Autodesk Fusion 360 part; units mm, degrees
note: some values were not read from the file. Set by a fixed rule: which sketch regions a step uses.
(part 16 of 20)
  spline S91 degree 5 poles (-29.6298, 9.1146) (-29.6276, 9.1129) (-29.6234, 9.1096) (-29.6169, 9.1047) (-29.6084, 9.0981) (-29.5977, 9.09) (-29.587, 9.0818) (-29.5763, 9.0737) (-29.5657, 9.0657) (-29.555, 9.0576) (-29.5444, 9.0496) (-29.5338, 9.0416) (-29.5232, 9.0337) (-29.5127, 9.0258) (-29.5021, 9.0179) (-29.4915, 9.0101) (-29.481, 9.0022) (-29.4705, 8.9945) (-29.46, 8.9867) (-29.4495, 8.979) (-29.4391, 8.9713) (-29.4286, 8.9637) (-29.4182, 8.956) (-29.4078, 8.9485) (-29.3974, 8.9409) (-29.387, 8.9334) (-29.3766, 8.9259) (-29.3663, 8.9184) (-29.356, 8.911) (-29.3457, 8.9036) (-29.3354, 8.8963) (-29.3251, 8.8889) (-29.3148, 8.8816) (-29.3046, 8.8744) (-29.2944, 8.8671) (-29.2842, 8.86) (-29.274, 8.8528) (-29.2638, 8.8457) (-29.2537, 8.8386) (-29.2435, 8.8315) (-29.2334, 8.8245) (-29.2233, 8.8175) (-29.2132, 8.8105) (-29.2032, 8.8036) (-29.1932, 8.7967) (-29.1831, 8.7898) (-29.1731, 8.783) (-29.1632, 8.7762) (-29.1532, 8.7694) (-29.1433, 8.7626) (-29.1334, 8.7559) (-29.1235, 8.7493) (-29.1136, 8.7426) (-29.1037, 8.736) (-29.0939, 8.7295) (-29.0841, 8.7229) (-29.0743, 8.7164) (-29.0646, 8.7099) (-29.0548, 8.7035) (-29.0451, 8.6971) (-29.0354, 8.6907) (-29.0257, 8.6844) (-29.016, 8.6781) (-29.0064, 8.6718) (-28.9968, 8.6656) (-28.9872, 8.6593) (-28.9776, 8.6532) (-28.9681, 8.647) (-28.9586, 8.6409) (-28.9491, 8.6348) (-28.9396, 8.6288) (-28.9302, 8.6228) (-28.9207, 8.6168) (-28.9113, 8.6109) (-28.902, 8.605) (-28.8926, 8.5991) (-28.8833, 8.5932) (-28.874, 8.5874) (-28.8647, 8.5817) (-28.8555, 8.5759) (-28.8462, 8.5702) (-28.837, 8.5645) (-28.8279, 8.5589) (-28.8187, 8.5533) (-28.8096, 8.5477) (-28.8005, 8.5422) (-28.7914, 8.5367) (-28.7824, 8.5312) (-28.7734, 8.5257) (-28.7644, 8.5203) (-28.7554, 8.515) (-28.7465, 8.5096) (-28.7376, 8.5043) (-28.7287, 8.499) (-28.7199, 8.4938) (-28.711, 8.4886) (-28.7022, 8.4834) (-28.6935, 8.4783) (-28.6847, 8.4732) (-28.676, 8.4681) (-28.6674, 8.463) (-28.6587, 8.458) (-28.6501, 8.4531) (-28.6415, 8.4481) (-28.633, 8.4432) (-28.6244, 8.4384) (-28.616, 8.4335) (-28.6075, 8.4287) (-28.5991, 8.4239) (-28.5907, 8.4192) (-28.5823, 8.4145) (-28.574, 8.4098) (-28.5657, 8.4052) (-28.5574, 8.4006) (-28.5491, 8.396) (-28.5409, 8.3915) (-28.5328, 8.387) (-28.5246, 8.3825) (-28.5165, 8.3781) (-28.5085, 8.3737) (-28.5004, 8.3693) (-28.4924, 8.365) (-28.4845, 8.3607) (-28.4765, 8.3565) (-28.4686, 8.3522) (-28.4608, 8.348) (-28.4529, 8.3439) (-28.4452, 8.3398) (-28.4374, 8.3357) (-28.4297, 8.3316) (-28.422, 8.3276) (-28.4144, 8.3236) (-28.4068, 8.3196) (-28.3992, 8.3157) (-28.3917, 8.3118) (-28.3842, 8.308) (-28.3767, 8.3042) (-28.3693, 8.3004) (-28.3619, 8.2966) (-28.3546, 8.2929) (-28.3473, 8.2892) (-28.3401, 8.2856) (-28.3329, 8.282) (-28.3257, 8.2784) (-28.3186, 8.2748) (-28.3115, 8.2713) (-28.3044, 8.2678) (-28.2974, 8.2644) (-28.2905, 8.261) (-28.2835, 8.2576) (-28.2767, 8.2543) (-28.2698, 8.251) (-28.263, 8.2477) (-28.2563, 8.2445) (-28.2496, 8.2412) (-28.2429, 8.2381) (-28.2363, 8.2349) (-28.2298, 8.2318) (-28.2233, 8.2288) (-28.2168, 8.2257) (-28.2104, 8.2227) (-28.204, 8.2198) (-28.1977, 8.2169) (-28.1914, 8.214) (-28.1851, 8.2111) (-28.179, 8.2083) (-28.1728, 8.2055) (-28.1667, 8.2027) (-28.1607, 8.2) (-28.1547, 8.1973) (-28.1488, 8.1947) (-28.1429, 8.192) (-28.1371, 8.1895) (-28.1313, 8.1869) (-28.1256, 8.1844) (-28.1199, 8.1819) (-28.1143, 8.1795) (-28.1087, 8.177) (-28.1032, 8.1747) (-28.0978, 8.1723) (-28.0924, 8.17) (-28.087, 8.1677) (-28.0818, 8.1655) (-28.0765, 8.1633) (-28.0714, 8.1611) (-28.0663, 8.159) (-28.0612, 8.1569) (-28.0562, 8.1548) (-28.0513, 8.1528) (-28.0464, 8.1508) (-28.0416, 8.1488) (-28.0369, 8.1469) (-28.0322, 8.145) (-28.0276, 8.1432) (-28.023, 8.1413) (-28.0185, 8.1395) (-28.0141, 8.1378) (-28.0097, 8.1361) (-28.0054, 8.1344) (-28.0012, 8.1327) (-27.997, 8.1311) (-27.9929, 8.1295) (-27.9889, 8.128) (-27.9849, 8.1265) (-27.9811, 8.125) (-27.9772, 8.1236) (-27.9735, 8.1222) (-27.9698, 8.1208) (-27.9662, 8.1194) (-27.9627, 8.1181) (-27.9593, 8.1169) (-27.9559, 8.1156) (-27.9526, 8.1144) (-27.9494, 8.1133) (-27.9462, 8.1121) (-27.9432, 8.1111) (-27.9402, 8.11) (-27.9373, 8.109) (-27.9345, 8.108) (-27.9318, 8.107) (-27.9291, 8.1061) (-27.9265, 8.1052) (-27.9241, 8.1044) (-27.9217, 8.1036) (-27.9194, 8.1028) (-27.9172, 8.102) (-27.915, 8.1013) (-27.913, 8.1007) (-27.9111, 8.1) (-27.9092, 8.0994) (-27.9075, 8.0988) (-27.9058, 8.0983) (-27.9043, 8.0978) (-27.9028, 8.0973) (-27.9015, 8.0969) (-27.9002, 8.0965) (-27.8991, 8.0962) (-27.898, 8.0958) (-27.8971, 8.0956) (-27.8963, 8.0953) (-27.8956, 8.0951) (-27.8951, 8.0949) (-27.8948, 8.0948) (-27.8946, 8.0948) (-27.8945, 8.0948) knots -1 -1 -1 -1 -1 -1 -0.99583333 -0.99166667 -0.9875 -0.98333333 -0.97916667 -0.975 -0.97083333 -0.96666667 -0.9625 -0.95833333 -0.95416667 -0.95 -0.94583333 -0.94166667 -0.9375 -0.93333333 -0.92916667 -0.925 -0.92083333 -0.91666667 -0.9125 -0.90833333 -0.90416667 -0.9 -0.89583333 -0.89166667 -0.8875 -0.88333333 -0.87916667 -0.875 -0.87083333 -0.86666667 -0.8625 -0.85833333 -0.85416667 -0.85 -0.84583333 -0.84166667 -0.8375 -0.83333333 -0.82916667 -0.825 -0.82083333 -0.81666667 -0.8125 -0.80833333 -0.80416667 -0.8 -0.79583333 -0.79166667 -0.7875 -0.78333333 -0.77916667 -0.775 -0.77083333 -0.76666667 -0.7625 -0.75833333 -0.75416667 -0.75 -0.74583333 -0.74166667 -0.7375 -0.73333333 -0.72916667 -0.725 -0.72083333 -0.71666667 -0.7125 -0.70833333 -0.70416667 -0.7 -0.69583333 -0.69166667 -0.6875 -0.68333333 -0.67916667 -0.675 -0.67083333 -0.66666667 -0.6625 -0.65833333 -0.65416667 -0.65 -0.64583333 -0.64166667 -0.6375 -0.63333333 -0.62916667 -0.625 -0.62083333 -0.61666667 -0.6125 -0.60833333 -0.60416667 -0.6 -0.59583333 -0.59166667 -0.5875 -0.58333333 -0.57916667 -0.575 -0.57083333 -0.56666667 -0.5625 -0.55833333 -0.55416667 -0.55 -0.54583333 -0.54166667 -0.5375 -0.53333333 -0.52916667 -0.525 -0.52083333 -0.51666667 -0.5125 -0.50833333 -0.50416667 -0.5 -0.49583333 -0.49166667 -0.4875 -0.48333333 -0.47916667 -0.475 -0.47083333 -0.46666667 -0.4625 -0.45833333 -0.45416667 -0.45 -0.44583333 -0.44166667 -0.4375 -0.43333333 -0.42916667 -0.425 -0.42083333 -0.41666667 -0.4125 -0.40833333 -0.40416667 -0.4 -0.39583333 -0.39166667 -0.3875 -0.38333333 -0.37916667 -0.375 -0.37083333 -0.36666667 -0.3625 -0.35833333 -0.35416667 -0.35 -0.34583333 -0.34166667 -0.3375 -0.33333333 -0.32916667 -0.325 -0.32083333 -0.31666667 -0.3125 -0.30833333 -0.30416667 -0.3 -0.29583333 -0.29166667 -0.2875 -0.28333333 -0.27916667 -0.275 -0.27083333 -0.26666667 -0.2625 -0.25833333 -0.25416667 -0.25 -0.24583333 -0.24166667 -0.2375 -0.23333333 -0.22916667 -0.225 -0.22083333 -0.21666667 -0.2125 -0.20833333 -0.20416667 -0.2 -0.19583333 -0.19166667 -0.1875 -0.18333333 -0.17916667 -0.175 -0.17083333 -0.16666667 -0.1625 -0.15833333 -0.15416667 -0.15 -0.14583333 -0.14166667 -0.1375 -0.13333333 -0.12916667 -0.125 -0.12083333 -0.11666667 -0.1125 -0.10833333 -0.10416667 -0.1 -0.09583333 -0.09166667 -0.0875 -0.08333333 -0.07916667 -0.075 -0.07083333 -0.06666667 -0.0625 -0.05833333 -0.05416667 -0.05 -0.04583333 -0.04166667 -0.0375 -0.03333333 -0.02916667 -0.025 -0.02083333 -0.01666667 -0.0125 -0.00833333 -0.00416667 0 0 0 0 0 0
  line L187 (-26.8955, 10.9662) -> (-26.8948, 10.9659)
  arc A90 (5.0824, 28.2972) -> (3.9106, 28.4828) centre (0, 0) ccw
  line L188 (-25.8803, 12.5209) -> (-26.1453, 12.6491)
  arc A91 (6.9214, 30.2174) -> (5.9675, 30.4202) centre (0, 0) ccw
  arc A92 (8.0125, 27.6109) -> (6.8665, 27.918) centre (0, 0) ccw
  line L189 (5.1345, 28.587) -> (5.0824, 28.2972)
  spline S92 degree 5 poles (9.1146, 29.6298) (9.1129, 29.6276) (9.1096, 29.6234) (9.1047, 29.6169) (9.0981, 29.6084) (9.09, 29.5977) (9.0818, 29.587) (9.0737, 29.5763) (9.0657, 29.5657) (9.0576, 29.555) (9.0496, 29.5444) (9.0416, 29.5338) (9.0337, 29.5232) (9.0258, 29.5127) (9.0179, 29.5021) (9.0101, 29.4915) (9.0022, 29.481) (8.9945, 29.4705) (8.9867, 29.46) (8.979, 29.4495) (8.9713, 29.4391) (8.9637, 29.4286) (8.956, 29.4182) (8.9485, 29.4078) (8.9409, 29.3974) (8.9334, 29.387) (8.9259, 29.3766) (8.9184, 29.3663) (8.911, 29.356) (8.9036, 29.3457) (8.8963, 29.3354) (8.8889, 29.3251) (8.8816, 29.3148) (8.8744, 29.3046) (8.8671, 29.2944) (8.86, 29.2842) (8.8528, 29.274) (8.8457, 29.2638) (8.8386, 29.2537) (8.8315, 29.2435) (8.8245, 29.2334) (8.8175, 29.2233) (8.8105, 29.2132) (8.8036, 29.2032) (8.7967, 29.1932) (8.7898, 29.1831) (8.783, 29.1731) (8.7762, 29.1632) (8.7694, 29.1532) (8.7626, 29.1433) (8.7559, 29.1334) (8.7493, 29.1235) (8.7426, 29.1136) (8.736, 29.1037) (8.7295, 29.0939) (8.7229, 29.0841) (8.7164, 29.0743) (8.7099, 29.0646) (8.7035, 29.0548) (8.6971, 29.0451) (8.6907, 29.0354) (8.6844, 29.0257) (8.6781, 29.016) (8.6718, 29.0064) (8.6656, 28.9968) (8.6593, 28.9872) (8.6532, 28.9776) (8.647, 28.9681) (8.6409, 28.9586) (8.6348, 28.9491) (8.6288, 28.9396) (8.6228, 28.9302) (8.6168, 28.9207) (8.6109, 28.9113) (8.605, 28.902) (8.5991, 28.8926) (8.5932, 28.8833) (8.5874, 28.874) (8.5817, 28.8647) (8.5759, 28.8555) (8.5702, 28.8462) (8.5645, 28.837) (8.5589, 28.8279) (8.5533, 28.8187) (8.5477, 28.8096) (8.5422, 28.8005) (8.5367, 28.7914) (8.5312, 28.7824) (8.5257, 28.7734) (8.5203, 28.7644) (8.515, 28.7554) (8.5096, 28.7465) (8.5043, 28.7376) (8.499, 28.7287) (8.4938, 28.7199) (8.4886, 28.711) (8.4834, 28.7022) (8.4783, 28.6935) (8.4732, 28.6847) (8.4681, 28.676) (8.463, 28.6674) (8.458, 28.6587) (8.4531, 28.6501) (8.4481, 28.6415) (8.4432, 28.633) (8.4384, 28.6244) (8.4335, 28.616) (8.4287, 28.6075) (8.4239, 28.5991) (8.4192, 28.5907) (8.4145, 28.5823) (8.4098, 28.574) (8.4052, 28.5657) (8.4006, 28.5574) (8.396, 28.5491) (8.3915, 28.5409) (8.387, 28.5328) (8.3825, 28.5246) (8.3781, 28.5165) (8.3737, 28.5085) (8.3693, 28.5004) (8.365, 28.4924) (8.3607, 28.4845) (8.3565, 28.4765) (8.3522, 28.4686) (8.348, 28.4608) (8.3439, 28.4529) (8.3398, 28.4452) (8.3357, 28.4374) (8.3316, 28.4297) (8.3276, 28.422) (8.3236, 28.4144) (8.3196, 28.4068) (8.3157, 28.3992) (8.3118, 28.3917) (8.308, 28.3842) (8.3042, 28.3767) (8.3004, 28.3693) (8.2966, 28.3619) (8.2929, 28.3546) (8.2892, 28.3473) (8.2856, 28.3401) (8.282, 28.3329) (8.2784, 28.3257) (8.2748, 28.3186) (8.2713, 28.3115) (8.2678, 28.3044) (8.2644, 28.2974) (8.261, 28.2905) (8.2576, 28.2835) (8.2543, 28.2767) (8.251, 28.2698) (8.2477, 28.263) (8.2445, 28.2563) (8.2412, 28.2496) (8.2381, 28.2429) (8.2349, 28.2363) (8.2318, 28.2298) (8.2288, 28.2233) (8.2257, 28.2168) (8.2227, 28.2104) (8.2198, 28.204) (8.2169, 28.1977) (8.214, 28.1914) (8.2111, 28.1851) (8.2083, 28.179) (8.2055, 28.1728) (8.2027, 28.1667) (8.2, 28.1607) (8.1973, 28.1547) (8.1947, 28.1488) (8.192, 28.1429) (8.1895, 28.1371) (8.1869, 28.1313) (8.1844, 28.1256) (8.1819, 28.1199) (8.1795, 28.1143) (8.177, 28.1087) (8.1747, 28.1032) (8.1723, 28.0978) (8.17, 28.0924) (8.1677, 28.087) (8.1655, 28.0818) (8.1633, 28.0765) (8.1611, 28.0714) (8.159, 28.0663) (8.1569, 28.0612) (8.1548, 28.0562) (8.1528, 28.0513) (8.1508, 28.0464) (8.1488, 28.0416) (8.1469, 28.0369) (8.145, 28.0322) (8.1432, 28.0276) (8.1413, 28.023) (8.1395, 28.0185) (8.1378, 28.0141) (8.1361, 28.0097) (8.1344, 28.0054) (8.1327, 28.0012) (8.1311, 27.997) (8.1295, 27.9929) (8.128, 27.9889) (8.1265, 27.9849) (8.125, 27.9811) (8.1236, 27.9772) (8.1222, 27.9735) (8.1208, 27.9698) (8.1194, 27.9662) (8.1181, 27.9627) (8.1169, 27.9593) (8.1156, 27.9559) (8.1144, 27.9526) (8.1133, 27.9494) (8.1121, 27.9462) (8.1111, 27.9432) (8.11, 27.9402) (8.109, 27.9373) (8.108, 27.9345) (8.107, 27.9318) (8.1061, 27.9291) (8.1052, 27.9265) (8.1044, 27.9241) (8.1036, 27.9217) (8.1028, 27.9194) (8.102, 27.9172) (8.1013, 27.915) (8.1007, 27.913) (8.1, 27.9111) (8.0994, 27.9092) (8.0988, 27.9075) (8.0983, 27.9058) (8.0978, 27.9043) (8.0973, 27.9028) (8.0969, 27.9015) (8.0965, 27.9002) (8.0962, 27.8991) (8.0958, 27.898) (8.0956, 27.8971) (8.0953, 27.8963) (8.0951, 27.8956) (8.0949, 27.8951) (8.0948, 27.8948) (8.0948, 27.8946) (8.0948, 27.8945) knots -1 -1 -1 -1 -1 -1 -0.99583333 -0.99166667 -0.9875 -0.98333333 -0.97916667 -0.975 -0.97083333 -0.96666667 -0.9625 -0.95833333 -0.95416667 -0.95 -0.94583333 -0.94166667 -0.9375 -0.93333333 -0.92916667 -0.925 -0.92083333 -0.91666667 -0.9125 -0.90833333 -0.90416667 -0.9 -0.89583333 -0.89166667 -0.8875 -0.88333333 -0.87916667 -0.875 -0.87083333 -0.86666667 -0.8625 -0.85833333 -0.85416667 -0.85 -0.84583333 -0.84166667 -0.8375 -0.83333333 -0.82916667 -0.825 -0.82083333 -0.81666667 -0.8125 -0.80833333 -0.80416667 -0.8 -0.79583333 -0.79166667 -0.7875 -0.78333333 -0.77916667 -0.775 -0.77083333 -0.76666667 -0.7625 -0.75833333 -0.75416667 -0.75 -0.74583333 -0.74166667 -0.7375 -0.73333333 -0.72916667 -0.725 -0.72083333 -0.71666667 -0.7125 -0.70833333 -0.70416667 -0.7 -0.69583333 -0.69166667 -0.6875 -0.68333333 -0.67916667 -0.675 -0.67083333 -0.66666667 -0.6625 -0.65833333 -0.65416667 -0.65 -0.64583333 -0.64166667 -0.6375 -0.63333333 -0.62916667 -0.625 -0.62083333 -0.61666667 -0.6125 -0.60833333 -0.60416667 -0.6 -0.59583333 -0.59166667 -0.5875 -0.58333333 -0.57916667 -0.575 -0.57083333 -0.56666667 -0.5625 -0.55833333 -0.55416667 -0.55 -0.54583333 -0.54166667 -0.5375 -0.53333333 -0.52916667 -0.525 -0.52083333 -0.51666667 -0.5125 -0.50833333 -0.50416667 -0.5 -0.49583333 -0.49166667 -0.4875 -0.48333333 -0.47916667 -0.475 -0.47083333 -0.46666667 -0.4625 -0.45833333 -0.45416667 -0.45 -0.44583333 -0.44166667 -0.4375 -0.43333333 -0.42916667 -0.425 -0.42083333 -0.41666667 -0.4125 -0.40833333 -0.40416667 -0.4 -0.39583333 -0.39166667 -0.3875 -0.38333333 -0.37916667 -0.375 -0.37083333 -0.36666667 -0.3625 -0.35833333 -0.35416667 -0.35 -0.34583333 -0.34166667 -0.3375 -0.33333333 -0.32916667 -0.325 -0.32083333 -0.31666667 -0.3125 -0.30833333 -0.30416667 -0.3 -0.29583333 -0.29166667 -0.2875 -0.28333333 -0.27916667 -0.275 -0.27083333 -0.26666667 -0.2625 -0.25833333 -0.25416667 -0.25 -0.24583333 -0.24166667 -0.2375 -0.23333333 -0.22916667 -0.225 -0.22083333 -0.21666667 -0.2125 -0.20833333 -0.20416667 -0.2 -0.19583333 -0.19166667 -0.1875 -0.18333333 -0.17916667 -0.175 -0.17083333 -0.16666667 -0.1625 -0.15833333 -0.15416667 -0.15 -0.14583333 -0.14166667 -0.1375 -0.13333333 -0.12916667 -0.125 -0.12083333 -0.11666667 -0.1125 -0.10833333 -0.10416667 -0.1 -0.09583333 -0.09166667 -0.0875 -0.08333333 -0.07916667 -0.075 -0.07083333 -0.06666667 -0.0625 -0.05833333 -0.05416667 -0.05 -0.04583333 -0.04166667 -0.0375 -0.03333333 -0.02916667 -0.025 -0.02083333 -0.01666667 -0.0125 -0.00833333 -0.00416667 0 0 0 0 0 0
  line L190 (-26.1453, 12.6491) -> (-26.1461, 12.6495)
  arc A93 (-27.6109, 8.0125) -> (-27.918, 6.8665) centre (0, 0) ccw
  line L191 (6.9368, 28.2039) -> (6.937, 28.2047)
  arc A94 (-10.8547, -26.6221) -> (-9.7471, -27.0473) centre (0, 0) ccw
  arc A95 (28.7355, 0.9119) -> (28.6734, 2.0967) centre (0, 0) ccw
  spline S93 degree 5 poles (-12.1618, -28.5147) (-12.16, -28.5128) (-12.1562, -28.5089) (-12.1506, -28.503) (-12.1432, -28.4951) (-12.134, -28.4854) (-12.1248, -28.4756) (-12.1156, -28.4658) (-12.1065, -28.4561) (-12.0973, -28.4464) (-12.0883, -28.4366) (-12.0792, -28.4269) (-12.0702, -28.4172) (-12.0613, -28.4075) (-12.0523, -28.3978) (-12.0434, -28.3882) (-12.0345, -28.3785) (-12.0257, -28.3689) (-12.0169, -28.3593) (-12.0081, -28.3496) (-11.9994, -28.34) (-11.9907, -28.3305) (-11.982, -28.3209) (-11.9734, -28.3113) (-11.9648, -28.3018) (-11.9562, -28.2922) (-11.9477, -28.2827) (-11.9392, -28.2732) (-11.9307, -28.2637) (-11.9223, -28.2542) (-11.9139, -28.2447) (-11.9055, -28.2353) (-11.8972, -28.2259) (-11.8889, -28.2164) (-11.8807, -28.207) (-11.8724, -28.1976) (-11.8643, -28.1882) (-11.8561, -28.1789) (-11.848, -28.1695) (-11.8399, -28.1602) (-11.8318, -28.1509) (-11.8238, -28.1416) (-11.8158, -28.1323) (-11.8079, -28.123) (-11.8, -28.1137) (-11.7921, -28.1045) (-11.7843, -28.0953) (-11.7765, -28.0861) (-11.7687, -28.0769) (-11.7609, -28.0677) (-11.7532, -28.0585) (-11.7456, -28.0494) (-11.7379, -28.0403) (-11.7303, -28.0312) (-11.7228, -28.0221) (-11.7153, -28.013) (-11.7078, -28.0039) (-11.7003, -27.9949) (-11.6929, -27.9859) (-11.6855, -27.9769) (-11.6781, -27.9679) (-11.6708, -27.9589) (-11.6635, -27.95) (-11.6563, -27.9411) (-11.6491, -27.9322) (-11.6419, -27.9233) (-11.6348, -27.9144) (-11.6276, -27.9055) (-11.6206, -27.8967) (-11.6135, -27.8879) (-11.6065, -27.8791) (-11.5996, -27.8704) (-11.5927, -27.8616) (-11.5858, -27.8529) (-11.5789, -27.8442) (-11.5721, -27.8355) (-11.5653, -27.8268) (-11.5585, -27.8182) (-11.5518, -27.8096) (-11.5452, -27.801) (-11.5385, -27.7924) (-11.5319, -27.7838) (-11.5253, -27.7753) (-11.5188, -27.7668) (-11.5123, -27.7583) (-11.5058, -27.7498) (-11.4994, -27.7414) (-11.493, -27.733) (-11.4867, -27.7246) (-11.4803, -27.7162) (-11.4741, -27.7078) (-11.4678, -27.6995) (-11.4616, -27.6912) (-11.4554, -27.6829) (-11.4493, -27.6747) (-11.4432, -27.6665) (-11.4371, -27.6582) (-11.4311, -27.6501) (-11.4251, -27.6419) (-11.4192, -27.6338) (-11.4132, -27.6257) (-11.4074, -27.6176) (-11.4015, -27.6096) (-11.3957, -27.6015) (-11.3899, -27.5936) (-11.3842, -27.5856) (-11.3785, -27.5776) (-11.3728, -27.5697) (-11.3672, -27.5618) (-11.3616, -27.554) (-11.3561, -27.5462) (-11.3506, -27.5384) (-11.3451, -27.5306) (-11.3396, -27.5228) (-11.3342, -27.5151) (-11.3289, -27.5074) (-11.3235, -27.4998) (-11.3183, -27.4922) (-11.313, -27.4846) (-11.3078, -27.477) (-11.3026, -27.4695) (-11.2975, -27.462) (-11.2924, -27.4545) (-11.2873, -27.447) (-11.2823, -27.4396) (-11.2773, -27.4323) (-11.2723, -27.4249) (-11.2674, -27.4176) (-11.2625, -27.4103) (-11.2577, -27.4031) (-11.2529, -27.3958) (-11.2481, -27.3887) (-11.2434, -27.3815) (-11.2387, -27.3744) (-11.234, -27.3673) (-11.2294, -27.3603) (-11.2248, -27.3533) (-11.2203, -27.3463) (-11.2158, -27.3393) (-11.2113, -27.3324) (-11.2069, -27.3256) (-11.2025, -27.3187) (-11.1982, -27.3119) (-11.1939, -27.3052) (-11.1896, -27.2985) (-11.1854, -27.2918) (-11.1812, -27.2851) (-11.177, -27.2785) (-11.1729, -27.272) (-11.1688, -27.2654) (-11.1648, -27.259) (-11.1608, -27.2525) (-11.1568, -27.2461) (-11.1529, -27.2397) (-11.149, -27.2334) (-11.1451, -27.2271) (-11.1413, -27.2209) (-11.1376, -27.2147) (-11.1338, -27.2085) (-11.1301, -27.2024) (-11.1265, -27.1963) (-11.1229, -27.1903) (-11.1193, -27.1843) (-11.1158, -27.1784) (-11.1123, -27.1725) (-11.1088, -27.1666) (-11.1054, -27.1608) (-11.102, -27.155) (-11.0987, -27.1493) (-11.0954, -27.1436) (-11.0921, -27.138) (-11.0889, -27.1324) (-11.0857, -27.1269) (-11.0826, -27.1214) (-11.0795, -27.116) (-11.0764, -27.1106) (-11.0734, -27.1053) (-11.0704, -27.1) (-11.0675, -27.0948) (-11.0646, -27.0896) (-11.0617, -27.0845) (-11.0589, -27.0794) (-11.0561, -27.0744) (-11.0534, -27.0694) (-11.0507, -27.0645) (-11.048, -27.0597) (-11.0454, -27.0549) (-11.0428, -27.0501) (-11.0403, -27.0454) (-11.0378, -27.0408) (-11.0353, -27.0362) (-11.0329, -27.0317) (-11.0306, -27.0272) (-11.0282, -27.0228) (-11.0259, -27.0185) (-11.0237, -27.0142) (-11.0215, -27.01) (-11.0193, -27.0058) (-11.0172, -27.0017) (-11.0151, -26.9977) (-11.0131, -26.9937) (-11.0111, -26.9898) (-11.0091, -26.986) (-11.0072, -26.9822) (-11.0053, -26.9785) (-11.0035, -26.9748) (-11.0017, -26.9713) (-10.9999, -26.9678) (-10.9982, -26.9643) (-10.9966, -26.961) (-10.9949, -26.9577) (-10.9934, -26.9544) (-10.9918, -26.9513) (-10.9903, -26.9482) (-10.9889, -26.9452) (-10.9875, -26.9423) (-10.9861, -26.9394) (-10.9848, -26.9366) (-10.9835, -26.9339) (-10.9823, -26.9313) (-10.9811, -26.9288) (-10.9799, -26.9263) (-10.9788, -26.924) (-10.9778, -26.9217) (-10.9768, -26.9195) (-10.9758, -26.9173) (-10.9749, -26.9153) (-10.974, -26.9134) (-10.9731, -26.9115) (-10.9724, -26.9097) (-10.9716, -26.908) (-10.9709, -26.9065) (-10.9702, -26.905) (-10.9696, -26.9036) (-10.9691, -26.9023) (-10.9685, -26.9011) (-10.9681, -26.9) (-10.9676, -26.899) (-10.9672, -26.8981) (-10.9669, -26.8973) (-10.9666, -26.8966) (-10.9664, -26.8961) (-10.9663, -26.8958) (-10.9662, -26.8956) (-10.9662, -26.8955) knots -1 -1 -1 -1 -1 -1 -0.99583333 -0.99166667 -0.9875 -0.98333333 -0.97916667 -0.975 -0.97083333 -0.96666667 -0.9625 -0.95833333 -0.95416667 -0.95 -0.94583333 -0.94166667 -0.9375 -0.93333333 -0.92916667 -0.925 -0.92083333 -0.91666667 -0.9125 -0.90833333 -0.90416667 -0.9 -0.89583333 -0.89166667 -0.8875 -0.88333333 -0.87916667 -0.875 -0.87083333 -0.86666667 -0.8625 -0.85833333 -0.85416667 -0.85 -0.84583333 -0.84166667 -0.8375 -0.83333333 -0.82916667 -0.825 -0.82083333 -0.81666667 -0.8125 -0.80833333 -0.80416667 -0.8 -0.79583333 -0.79166667 -0.7875 -0.78333333 -0.77916667 -0.775 -0.77083333 -0.76666667 -0.7625 -0.75833333 -0.75416667 -0.75 -0.74583333 -0.74166667 -0.7375 -0.73333333 -0.72916667 -0.725 -0.72083333 -0.71666667 -0.7125 -0.70833333 -0.70416667 -0.7 -0.69583333 -0.69166667 -0.6875 -0.68333333 -0.67916667 -0.675 -0.67083333 -0.66666667 -0.6625 -0.65833333 -0.65416667 -0.65 -0.64583333 -0.64166667 -0.6375 -0.63333333 -0.62916667 -0.625 -0.62083333 -0.61666667 -0.6125 -0.60833333 -0.60416667 -0.6 -0.59583333 -0.59166667 -0.5875 -0.58333333 -0.57916667 -0.575 -0.57083333 -0.56666667 -0.5625 -0.55833333 -0.55416667 -0.55 -0.54583333 -0.54166667 -0.5375 -0.53333333 -0.52916667 -0.525 -0.52083333 -0.51666667 -0.5125 -0.50833333 -0.50416667 -0.5 -0.49583333 -0.49166667 -0.4875 -0.48333333 -0.47916667 -0.475 -0.47083333 -0.46666667 -0.4625 -0.45833333 -0.45416667 -0.45 -0.44583333 -0.44166667 -0.4375 -0.43333333 -0.42916667 -0.425 -0.42083333 -0.41666667 -0.4125 -0.40833333 -0.40416667 -0.4 -0.39583333 -0.39166667 -0.3875 -0.38333333 -0.37916667 -0.375 -0.37083333 -0.36666667 -0.3625 -0.35833333 -0.35416667 -0.35 -0.34583333 -0.34166667 -0.3375 -0.33333333 -0.32916667 -0.325 -0.32083333 -0.31666667 -0.3125 -0.30833333 -0.30416667 -0.3 -0.29583333 -0.29166667 -0.2875 -0.28333333 -0.27916667 -0.275 -0.27083333 -0.26666667 -0.2625 -0.25833333 -0.25416667 -0.25 -0.24583333 -0.24166667 -0.2375 -0.23333333 -0.22916667 -0.225 -0.22083333 -0.21666667 -0.2125 -0.20833333 -0.20416667 -0.2 -0.19583333 -0.19166667 -0.1875 -0.18333333 -0.17916667 -0.175 -0.17083333 -0.16666667 -0.1625 -0.15833333 -0.15416667 -0.15 -0.14583333 -0.14166667 -0.1375 -0.13333333 -0.12916667 -0.125 -0.12083333 -0.11666667 -0.1125 -0.10833333 -0.10416667 -0.1 -0.09583333 -0.09166667 -0.0875 -0.08333333 -0.07916667 -0.075 -0.07083333 -0.06666667 -0.0625 -0.05833333 -0.05416667 -0.05 -0.04583333 -0.04166667 -0.0375 -0.03333333 -0.02916667 -0.025 -0.02083333 -0.01666667 -0.0125 -0.00833333 -0.00416667 0 0 0 0 0 0
  line L192 (29.0298, 0.9213) -> (28.7355, 0.9119)
  arc A96 (-19.9055, 20.7445) -> (-20.7445, 19.9055) centre (0, 0) ccw
  spline S94 degree 5 poles (-9.8472, -27.3251) (-9.8472, -27.3252) (-9.8473, -27.3254) (-9.8474, -27.3257) (-9.8475, -27.3262) (-9.8478, -27.3269) (-9.8481, -27.3277) (-9.8484, -27.3286) (-9.8487, -27.3296) (-9.8491, -27.3308) (-9.8495, -27.332) (-9.85, -27.3334) (-9.8505, -27.3348) (-9.851, -27.3364) (-9.8515, -27.338) (-9.8521, -27.3398) (-9.8527, -27.3416) (-9.8533, -27.3435) (-9.8539, -27.3456) (-9.8546, -27.3477) (-9.8553, -27.3499) (-9.856, -27.3523) (-9.8568, -27.3547) (-9.8575, -27.3572) (-9.8583, -27.3598) (-9.8591, -27.3625) (-9.86, -27.3652) (-9.8608, -27.3681) (-9.8617, -27.371) (-9.8626, -27.3741) (-9.8635, -27.3772) (-9.8645, -27.3804) (-9.8654, -27.3837) (-9.8664, -27.387) (-9.8674, -27.3905) (-9.8684, -27.394) (-9.8694, -27.3976) (-9.8704, -27.4013) (-9.8715, -27.4051) (-9.8725, -27.409) (-9.8736, -27.4129) (-9.8747, -27.4169) (-9.8758, -27.421) (-9.8769, -27.4252) (-9.878, -27.4294) (-9.8792, -27.4337) (-9.8803, -27.4381) (-9.8815, -27.4426) (-9.8827, -27.4471) (-9.8838, -27.4517) (-9.885, -27.4564) (-9.8862, -27.4612) (-9.8874, -27.466) (-9.8887, -27.4709) (-9.8899, -27.4759) (-9.8911, -27.481) (-9.8924, -27.4861) (-9.8936, -27.4912) (-9.8949, -27.4965) (-9.8962, -27.5018) (-9.8974, -27.5072) (-9.8987, -27.5127) (-9.9, -27.5182) (-9.9013, -27.5238) (-9.9026, -27.5294) (-9.9039, -27.5352) (-9.9052, -27.5409) (-9.9065, -27.5468) (-9.9079, -27.5527) (-9.9092, -27.5587) (-9.9105, -27.5647) (-9.9118, -27.5709) (-9.9132, -27.577) (-9.9145, -27.5833) (-9.9158, -27.5896) (-9.9172, -27.5959) (-9.9185, -27.6023) (-9.9199, -27.6088) (-9.9212, -27.6154) (-9.9225, -27.622) (-9.9239, -27.6286) (-9.9252, -27.6353) (-9.9266, -27.6421) (-9.9279, -27.649) (-9.9293, -27.6559) (-9.9306, -27.6628) (-9.932, -27.6698) (-9.9333, -27.6769) (-9.9347, -27.6841) (-9.936, -27.6912) (-9.9374, -27.6985) (-9.9387, -27.7058) (-9.9401, -27.7132) (-9.9414, -27.7206) (-9.9428, -27.728) (-9.9441, -27.7356) (-9.9454, -27.7431) (-9.9468, -27.7508) (-9.9481, -27.7585) (-9.9494, -27.7662) (-9.9508, -27.774) (-9.9521, -27.7819) (-9.9534, -27.7898) (-9.9547, -27.7977) (-9.956, -27.8057) (-9.9573, -27.8138) (-9.9586, -27.8219) (-9.9599, -27.8301) (-9.9612, -27.8383) (-9.9625, -27.8466) (-9.9638, -27.8549) (-9.9651, -27.8633) (-9.9664, -27.8717) (-9.9676, -27.8802) (-9.9689, -27.8887) (-9.9701, -27.8973) (-9.9714, -27.9059) (-9.9726, -27.9146) (-9.9739, -27.9233) (-9.9751, -27.9321) (-9.9763, -27.9409) (-9.9776, -27.9498) (-9.9788, -27.9587) (-9.98, -27.9677) (-9.9812, -27.9767) (-9.9824, -27.9858) (-9.9836, -27.9949) (-9.9847, -28.004) (-9.9859, -28.0133) (-9.9871, -28.0225) (-9.9882, -28.0318) (-9.9894, -28.0412) (-9.9905, -28.0506) (-9.9916, -28.06) (-9.9928, -28.0695) (-9.9939, -28.079) (-9.995, -28.0886) (-9.9961, -28.0982) (-9.9972, -28.1079) (-9.9983, -28.1176) (-9.9993, -28.1274) (-10.0004, -28.1372) (-10.0014, -28.147) (-10.0025, -28.1569) (-10.0035, -28.1668) (-10.0045, -28.1768) (-10.0055, -28.1868) (-10.0065, -28.1969) (-10.0075, -28.207) (-10.0085, -28.2172) (-10.0095, -28.2274) (-10.0104, -28.2376) (-10.0114, -28.2479) (-10.0123, -28.2582) (-10.0133, -28.2686) (-10.0142, -28.279) (-10.0151, -28.2894) (-10.016, -28.2999) (-10.0169, -28.3105) (-10.0177, -28.321) (-10.0186, -28.3317) (-10.0195, -28.3423) (-10.0203, -28.353) (-10.0211, -28.3638) (-10.0219, -28.3745) (-10.0227, -28.3854) (-10.0235, -28.3962) (-10.0243, -28.4071) (-10.0251, -28.4181) (-10.0258, -28.429) (-10.0266, -28.44) (-10.0273, -28.4511) (-10.028, -28.4622) (-10.0287, -28.4733) (-10.0294, -28.4845) (-10.0301, -28.4957) (-10.0308, -28.507) (-10.0314, -28.5183) (-10.0321, -28.5296) (-10.0327, -28.541) (-10.0333, -28.5524) (-10.0339, -28.5638) (-10.0345, -28.5753) (-10.0351, -28.5868) (-10.0356, -28.5984) (-10.0362, -28.61) (-10.0367, -28.6216) (-10.0372, -28.6333) (-10.0377, -28.645) (-10.0382, -28.6567) (-10.0387, -28.6685) (-10.0392, -28.6803) (-10.0396, -28.6922) (-10.04, -28.7041) (-10.0405, -28.716) (-10.0409, -28.728) (-10.0412, -28.74) (-10.0416, -28.752) (-10.042, -28.7641) (-10.0423, -28.7762) (-10.0427, -28.7883) (-10.043, -28.8005) (-10.0433, -28.8127) (-10.0436, -28.8249) (-10.0438, -28.8372) (-10.0441, -28.8495) (-10.0443, -28.8619) (-10.0445, -28.8743) (-10.0448, -28.8867) (-10.0449, -28.8991) (-10.0451, -28.9116) (-10.0453, -28.9241) (-10.0454, -28.9367) (-10.0456, -28.9493) (-10.0457, -28.9619) (-10.0458, -28.9745) (-10.0458, -28.9872) (-10.0459, -29) (-10.046, -29.0127) (-10.046, -29.0255) (-10.046, -29.0383) (-10.046, -29.0512) (-10.046, -29.0641) (-10.046, -29.077) (-10.0459, -29.0899) (-10.0458, -29.1029) (-10.0458, -29.1159) (-10.0457, -29.129) (-10.0455, -29.142) (-10.0454, -29.1551) (-10.0453, -29.1683) (-10.0451, -29.1815) (-10.0449, -29.1947) (-10.0447, -29.2079) (-10.0445, -29.2212) (-10.0442, -29.2345) (-10.044, -29.2478) (-10.0437, -29.2612) (-10.0434, -29.2745) (-10.0431, -29.288) (-10.0428, -29.3014) (-10.0425, -29.3122) (-10.0423, -29.3203) (-10.0422, -29.3257) (-10.0421, -29.3284) knots 0 0 0 0 0 0 0.00416667 0.00833333 0.0125 0.01666667 0.02083333 0.025 0.02916667 0.03333333 0.0375 0.04166667 0.04583333 0.05 0.05416667 0.05833333 0.0625 0.06666667 0.07083333 0.075 0.07916667 0.08333333 0.0875 0.09166667 0.09583333 0.1 0.10416667 0.10833333 0.1125 0.11666667 0.12083333 0.125 0.12916667 0.13333333 0.1375 0.14166667 0.14583333 0.15 0.15416667 0.15833333 0.1625 0.16666667 0.17083333 0.175 0.17916667 0.18333333 0.1875 0.19166667 0.19583333 0.2 0.20416667 0.20833333 0.2125 0.21666667 0.22083333 0.225 0.22916667 0.23333333 0.2375 0.24166667 0.24583333 0.25 0.25416667 0.25833333 0.2625 0.26666667 0.27083333 0.275 0.27916667 0.28333333 0.2875 0.29166667 0.29583333 0.3 0.30416667 0.30833333 0.3125 0.31666667 0.32083333 0.325 0.32916667 0.33333333 0.3375 0.34166667 0.34583333 0.35 0.35416667 0.35833333 0.3625 0.36666667 0.37083333 0.375 0.37916667 0.38333333 0.3875 0.39166667 0.39583333 0.4 0.40416667 0.40833333 0.4125 0.41666667 0.42083333 0.425 0.42916667 0.43333333 0.4375 0.44166667 0.44583333 0.45 0.45416667 0.45833333 0.4625 0.46666667 0.47083333 0.475 0.47916667 0.48333333 0.4875 0.49166667 0.49583333 0.5 0.50416667 0.50833333 0.5125 0.51666667 0.52083333 0.525 0.52916667 0.53333333 0.5375 0.54166667 0.54583333 0.55 0.55416667 0.55833333 0.5625 0.56666667 0.57083333 0.575 0.57916667 0.58333333 0.5875 0.59166667 0.59583333 0.6 0.60416667 0.60833333 0.6125 0.61666667 0.62083333 0.625 0.62916667 0.63333333 0.6375 0.64166667 0.64583333 0.65 0.65416667 0.65833333 0.6625 0.66666667 0.67083333 0.675 0.67916667 0.68333333 0.6875 0.69166667 0.69583333 0.7 0.70416667 0.70833333 0.7125 0.71666667 0.72083333 0.725 0.72916667 0.73333333 0.7375 0.74166667 0.74583333 0.75 0.75416667 0.75833333 0.7625 0.76666667 0.77083333 0.775 0.77916667 0.78333333 0.7875 0.79166667 0.79583333 0.8 0.80416667 0.80833333 0.8125 0.81666667 0.82083333 0.825 0.82916667 0.83333333 0.8375 0.84166667 0.84583333 0.85 0.85416667 0.85833333 0.8625 0.86666667 0.87083333 0.875 0.87916667 0.88333333 0.8875 0.89166667 0.89583333 0.9 0.90416667 0.90833333 0.9125 0.91666667 0.92083333 0.925 0.92916667 0.93333333 0.9375 0.94166667 0.94583333 0.95 0.95416667 0.95833333 0.9625 0.96666667 0.97083333 0.975 0.97916667 0.98333333 0.9875 0.99166667 0.99583333 1 1 1 1 1 1
  circle A97 centre (0, -10) radius 1.7
  line L193 (28.587, 5.1345) -> (28.5878, 5.1346)
  spline S95 degree 5 poles (28.9679, 2.1183) (28.968, 2.1183) (28.9682, 2.1183) (28.9685, 2.1183) (28.969, 2.1184) (28.9698, 2.1184) (28.9706, 2.1185) (28.9716, 2.1186) (28.9727, 2.1187) (28.9739, 2.1188) (28.9752, 2.1189) (28.9766, 2.1191) (28.9781, 2.1192) (28.9798, 2.1194) (28.9815, 2.1196) (28.9833, 2.1198) (28.9852, 2.12) (28.9873, 2.1202) (28.9894, 2.1204) (28.9916, 2.1207) (28.9939, 2.121) (28.9963, 2.1212) (28.9989, 2.1215) (29.0015, 2.1219) (29.0041, 2.1222) (29.0069, 2.1225) (29.0098, 2.1229) (29.0128, 2.1233) (29.0158, 2.1237) (29.0189, 2.1241) (29.0222, 2.1245) (29.0255, 2.125) (29.0289, 2.1254) (29.0323, 2.1259) (29.0359, 2.1264) (29.0395, 2.127) (29.0432, 2.1275) (29.047, 2.1281) (29.0509, 2.1286) (29.0549, 2.1292) (29.0589, 2.1299) (29.063, 2.1305) (29.0672, 2.1312) (29.0714, 2.1318) (29.0758, 2.1325) (29.0802, 2.1332) (29.0847, 2.134) (29.0892, 2.1347) (29.0938, 2.1355) (29.0985, 2.1363) (29.1033, 2.1371) (29.1081, 2.138) (29.1131, 2.1388) (29.118, 2.1397) (29.1231, 2.1406) (29.1282, 2.1415) (29.1334, 2.1424) (29.1386, 2.1434) (29.1439, 2.1444) (29.1493, 2.1454) (29.1547, 2.1464) (29.1602, 2.1475) (29.1658, 2.1485) (29.1714, 2.1496) (29.1771, 2.1507) (29.1829, 2.1519) (29.1887, 2.153) (29.1946, 2.1542) (29.2005, 2.1554) (29.2065, 2.1567) (29.2126, 2.1579) (29.2187, 2.1592) (29.2249, 2.1605) (29.2311, 2.1618) (29.2374, 2.1631) (29.2438, 2.1645) (29.2502, 2.1659) (29.2567, 2.1673) (29.2632, 2.1687) (29.2698, 2.1702) (29.2764, 2.1716) (29.2831, 2.1731) (29.2899, 2.1747) (29.2967, 2.1762) (29.3035, 2.1778) (29.3104, 2.1794) (29.3174, 2.181) (29.3244, 2.1827) (29.3314, 2.1843) (29.3386, 2.186) (29.3457, 2.1877) (29.3529, 2.1895) (29.3602, 2.1912) (29.3675, 2.193) (29.3749, 2.1948) (29.3823, 2.1967) (29.3898, 2.1985) (29.3973, 2.2004) (29.4049, 2.2023) (29.4125, 2.2043) (29.4202, 2.2062) (29.4279, 2.2082) (29.4356, 2.2102) (29.4434, 2.2123) (29.4513, 2.2143) (29.4592, 2.2164) (29.4671, 2.2185) (29.4751, 2.2207) (29.4832, 2.2228) (29.4912, 2.225) (29.4994, 2.2272) (29.5075, 2.2295) (29.5158, 2.2317) (29.524, 2.234) (29.5323, 2.2363) (29.5407, 2.2387) (29.5491, 2.241) (29.5575, 2.2434) (29.566, 2.2458) (29.5745, 2.2483) (29.583, 2.2508) (29.5917, 2.2533) (29.6003, 2.2558) (29.609, 2.2583) (29.6177, 2.2609) (29.6265, 2.2635) (29.6353, 2.2661) (29.6441, 2.2688) (29.653, 2.2714) (29.6619, 2.2741) (29.6709, 2.2769) (29.6799, 2.2796) (29.689, 2.2824) (29.6981, 2.2852) (29.7072, 2.288) (29.7163, 2.2909) (29.7255, 2.2938) (29.7348, 2.2967) (29.7441, 2.2996) (29.7534, 2.3026) (29.7627, 2.3056) (29.7721, 2.3086) (29.7815, 2.3117) (29.791, 2.3147) (29.8005, 2.3178) (29.81, 2.321) (29.8196, 2.3241) (29.8292, 2.3273) (29.8388, 2.3305) (29.8485, 2.3337) (29.8582, 2.337) (29.868, 2.3403) (29.8777, 2.3436) (29.8875, 2.3469) (29.8974, 2.3503) (29.9073, 2.3537) (29.9172, 2.3571) (29.9271, 2.3606) (29.9371, 2.364) (29.9471, 2.3675) (29.9572, 2.3711) (29.9673, 2.3746) (29.9774, 2.3782) (29.9875, 2.3818) (29.9977, 2.3855) (30.0079, 2.3891) (30.0182, 2.3928) (30.0284, 2.3965) (30.0388, 2.4003) (30.0491, 2.4041) (30.0595, 2.4079) (30.0699, 2.4117) (30.0803, 2.4156) (30.0907, 2.4194) (30.1012, 2.4234) (30.1118, 2.4273) (30.1223, 2.4313) (30.1329, 2.4353) (30.1435, 2.4393) (30.1541, 2.4433) (30.1648, 2.4474) (30.1755, 2.4515) (30.1862, 2.4557) (30.197, 2.4598) (30.2078, 2.464) (30.2186, 2.4682) (30.2294, 2.4725) (30.2403, 2.4767) (30.2512, 2.481) (30.2621, 2.4854) (30.2731, 2.4897) (30.2841, 2.4941) (30.2951, 2.4985) (30.3061, 2.503) (30.3172, 2.5074) (30.3283, 2.5119) (30.3394, 2.5165) (30.3506, 2.521) (30.3617, 2.5256) (30.3729, 2.5302) (30.3841, 2.5348) (30.3954, 2.5395) (30.4067, 2.5442) (30.418, 2.5489) (30.4293, 2.5537) (30.4407, 2.5584) (30.452, 2.5632) (30.4634, 2.5681) (30.4749, 2.5729) (30.4863, 2.5778) (30.4978, 2.5827) (30.5093, 2.5877) (30.5208, 2.5927) (30.5324, 2.5977) (30.5439, 2.6027) (30.5555, 2.6077) (30.5672, 2.6128) (30.5788, 2.6179) (30.5905, 2.6231) (30.6022, 2.6283) (30.6139, 2.6335) (30.6256, 2.6387) (30.6374, 2.6439) (30.6492, 2.6492) (30.661, 2.6545) (30.6728, 2.6599) (30.6847, 2.6653) (30.6966, 2.6707) (30.7085, 2.6761) (30.7204, 2.6815) (30.7323, 2.687) (30.7443, 2.6925) (30.7563, 2.6981) (30.7683, 2.7036) (30.7803, 2.7092) (30.7924, 2.7149) (30.8044, 2.7205) (30.8165, 2.7262) (30.8287, 2.7319) (30.8408, 2.7376) (30.853, 2.7434) (30.8627, 2.748) (30.87, 2.7515) (30.8749, 2.7539) (30.8773, 2.755) knots 0 0 0 0 0 0 0.00416667 0.00833333 0.0125 0.01666667 0.02083333 0.025 0.02916667 0.03333333 0.0375 0.04166667 0.04583333 0.05 0.05416667 0.05833333 0.0625 0.06666667 0.07083333 0.075 0.07916667 0.08333333 0.0875 0.09166667 0.09583333 0.1 0.10416667 0.10833333 0.1125 0.11666667 0.12083333 0.125 0.12916667 0.13333333 0.1375 0.14166667 0.14583333 0.15 0.15416667 0.15833333 0.1625 0.16666667 0.17083333 0.175 0.17916667 0.18333333 0.1875 0.19166667 0.19583333 0.2 0.20416667 0.20833333 0.2125 0.21666667 0.22083333 0.225 0.22916667 0.23333333 0.2375 0.24166667 0.24583333 0.25 0.25416667 0.25833333 0.2625 0.26666667 0.27083333 0.275 0.27916667 0.28333333 0.2875 0.29166667 0.29583333 0.3 0.30416667 0.30833333 0.3125 0.31666667 0.32083333 0.325 0.32916667 0.33333333 0.3375 0.34166667 0.34583333 0.35 0.35416667 0.35833333 0.3625 0.36666667 0.37083333 0.375 0.37916667 0.38333333 0.3875 0.39166667 0.39583333 0.4 0.40416667 0.40833333 0.4125 0.41666667 0.42083333 0.425 0.42916667 0.43333333 0.4375 0.44166667 0.44583333 0.45 0.45416667 0.45833333 0.4625 0.46666667 0.47083333 0.475 0.47916667 0.48333333 0.4875 0.49166667 0.49583333 0.5 0.50416667 0.50833333 0.5125 0.51666667 0.52083333 0.525 0.52916667 0.53333333 0.5375 0.54166667 0.54583333 0.55 0.55416667 0.55833333 0.5625 0.56666667 0.57083333 0.575 0.57916667 0.58333333 0.5875 0.59166667 0.59583333 0.6 0.60416667 0.60833333 0.6125 0.61666667 0.62083333 0.625 0.62916667 0.63333333 0.6375 0.64166667 0.64583333 0.65 0.65416667 0.65833333 0.6625 0.66666667 0.67083333 0.675 0.67916667 0.68333333 0.6875 0.69166667 0.69583333 0.7 0.70416667 0.70833333 0.7125 0.71666667 0.72083333 0.725 0.72916667 0.73333333 0.7375 0.74166667 0.74583333 0.75 0.75416667 0.75833333 0.7625 0.76666667 0.77083333 0.775 0.77916667 0.78333333 0.7875 0.79166667 0.79583333 0.8 0.80416667 0.80833333 0.8125 0.81666667 0.82083333 0.825 0.82916667 0.83333333 0.8375 0.84166667 0.84583333 0.85 0.85416667 0.85833333 0.8625 0.86666667 0.87083333 0.875 0.87916667 0.88333333 0.8875 0.89166667 0.89583333 0.9 0.90416667 0.90833333 0.9125 0.91666667 0.92083333 0.925 0.92916667 0.93333333 0.9375 0.94166667 0.94583333 0.95 0.95416667 0.95833333 0.9625 0.96666667 0.97083333 0.975 0.97916667 0.98333333 0.9875 0.99166667 0.99583333 1 1 1 1 1 1
  arc A98 (-21.9649, 18.5501) -> (-22.7115, 17.6281) centre (0, 0) ccw
  spline S96 degree 5 poles (-20.9575, 20.11) (-20.9576, 20.11) (-20.9577, 20.1102) (-20.958, 20.1104) (-20.9583, 20.1107) (-20.9589, 20.1112) (-20.9595, 20.1118) (-20.9602, 20.1125) (-20.961, 20.1132) (-20.9619, 20.114) (-20.9629, 20.1149) (-20.9639, 20.1159) (-20.9651, 20.1169) (-20.9663, 20.118) (-20.9675, 20.1192) (-20.9689, 20.1204) (-20.9704, 20.1217) (-20.9719, 20.123) (-20.9735, 20.1245) (-20.9752, 20.126) (-20.9769, 20.1275) (-20.9787, 20.1291) (-20.9806, 20.1308) (-20.9826, 20.1325) (-20.9847, 20.1343) (-20.9868, 20.1361) (-20.989, 20.138) (-20.9912, 20.1399) (-20.9936, 20.1419) (-20.996, 20.144) (-20.9984, 20.1461) (-21.001, 20.1482) (-21.0036, 20.1504) (-21.0063, 20.1527) (-21.009, 20.155) (-21.0119, 20.1573) (-21.0148, 20.1597) (-21.0177, 20.1622) (-21.0207, 20.1647) (-21.0238, 20.1672) (-21.027, 20.1698) (-21.0302, 20.1724) (-21.0335, 20.1751) (-21.0368, 20.1778) (-21.0403, 20.1806) (-21.0437, 20.1834) (-21.0473, 20.1862) (-21.0509, 20.1891) (-21.0546, 20.192) (-21.0583, 20.195) (-21.0621, 20.198) (-21.066, 20.201) (-21.0699, 20.2041) (-21.0739, 20.2072) (-21.0779, 20.2103) (-21.082, 20.2135) (-21.0862, 20.2167) (-21.0904, 20.22) (-21.0947, 20.2233) (-21.099, 20.2266) (-21.1034, 20.23) (-21.1079, 20.2333) (-21.1124, 20.2368) (-21.117, 20.2402) (-21.1216, 20.2437) (-21.1263, 20.2472) (-21.1311, 20.2508) (-21.1359, 20.2544) (-21.1408, 20.258) (-21.1457, 20.2616) (-21.1507, 20.2653) (-21.1557, 20.269) (-21.1608, 20.2727) (-21.166, 20.2765) (-21.1712, 20.2802) (-21.1764, 20.2841) (-21.1818, 20.2879) (-21.1871, 20.2918) (-21.1926, 20.2956) (-21.1981, 20.2996) (-21.2036, 20.3035) (-21.2092, 20.3075) (-21.2148, 20.3115) (-21.2205, 20.3155) (-21.2263, 20.3195) (-21.2321, 20.3236) (-21.238, 20.3277) (-21.2439, 20.3318) (-21.2498, 20.3359) (-21.2559, 20.3401) (-21.2619, 20.3442) (-21.2681, 20.3484) (-21.2742, 20.3527) (-21.2805, 20.3569) (-21.2867, 20.3612) (-21.2931, 20.3655) (-21.2995, 20.3698) (-21.3059, 20.3741) (-21.3124, 20.3784) (-21.3189, 20.3828) (-21.3255, 20.3872) (-21.3321, 20.3916) (-21.3388, 20.396) (-21.3455, 20.4004) (-21.3523, 20.4049) (-21.3592, 20.4094) (-21.3661, 20.4139) (-21.373, 20.4184) (-21.38, 20.4229) (-21.387, 20.4274) (-21.3941, 20.432) (-21.4012, 20.4366) (-21.4084, 20.4412) (-21.4156, 20.4458) (-21.4229, 20.4504) (-21.4302, 20.455) (-21.4376, 20.4597) (-21.445, 20.4644) (-21.4525, 20.469) (-21.46, 20.4737) (-21.4676, 20.4784) (-21.4752, 20.4832) (-21.4828, 20.4879) (-21.4905, 20.4927) (-21.4983, 20.4974) (-21.5061, 20.5022) (-21.5139, 20.507) (-21.5218, 20.5118) (-21.5297, 20.5166) (-21.5377, 20.5214) (-21.5458, 20.5263) (-21.5538, 20.5311) (-21.5619, 20.536) (-21.5701, 20.5409) (-21.5783, 20.5457) (-21.5866, 20.5506) (-21.5949, 20.5555) (-21.6032, 20.5605) (-21.6116, 20.5654) (-21.6201, 20.5703) (-21.6285, 20.5753) (-21.6371, 20.5802) (-21.6456, 20.5852) (-21.6542, 20.5902) (-21.6629, 20.5951) (-21.6716, 20.6001) (-21.6803, 20.6051) (-21.6891, 20.6101) (-21.698, 20.6152) (-21.7068, 20.6202) (-21.7158, 20.6252) (-21.7247, 20.6303) (-21.7337, 20.6353) (-21.7428, 20.6404) (-21.7519, 20.6454) (-21.761, 20.6505) (-21.7702, 20.6556) (-21.7794, 20.6607) (-21.7887, 20.6658) (-21.798, 20.6709) (-21.8073, 20.676) (-21.8167, 20.6811) (-21.8261, 20.6862) (-21.8356, 20.6913) (-21.8451, 20.6965) (-21.8547, 20.7016) (-21.8643, 20.7067) (-21.8739, 20.7119) (-21.8836, 20.717) (-21.8933, 20.7222) (-21.9031, 20.7274) (-21.9129, 20.7325) (-21.9228, 20.7377) (-21.9326, 20.7429) (-21.9426, 20.748) (-21.9525, 20.7532) (-21.9625, 20.7584) (-21.9726, 20.7636) (-21.9827, 20.7688) (-21.9928, 20.774) (-22.003, 20.7792) (-22.0132, 20.7844) (-22.0235, 20.7896) (-22.0337, 20.7948) (-22.0441, 20.8) (-22.0544, 20.8052) (-22.0649, 20.8105) (-22.0753, 20.8157) (-22.0858, 20.8209) (-22.0963, 20.8261) (-22.1069, 20.8313) (-22.1175, 20.8366) (-22.1281, 20.8418) (-22.1388, 20.847) (-22.1496, 20.8523) (-22.1603, 20.8575) (-22.1711, 20.8627) (-22.182, 20.868) (-22.1928, 20.8732) (-22.2038, 20.8784) (-22.2147, 20.8837) (-22.2257, 20.8889) (-22.2367, 20.8942) (-22.2478, 20.8994) (-22.2589, 20.9046) (-22.2701, 20.9099) (-22.2812, 20.9151) (-22.2925, 20.9204) (-22.3037, 20.9256) (-22.315, 20.9308) (-22.3264, 20.9361) (-22.3377, 20.9413) (-22.3491, 20.9466) (-22.3606, 20.9518) (-22.3721, 20.957) (-22.3836, 20.9623) (-22.3951, 20.9675) (-22.4067, 20.9727) (-22.4184, 20.978) (-22.43, 20.9832) (-22.4417, 20.9884) (-22.4535, 20.9937) (-22.4653, 20.9989) (-22.4771, 21.0041) (-22.4889, 21.0093) (-22.5008, 21.0145) (-22.5127, 21.0198) (-22.5247, 21.025) (-22.5367, 21.0302) (-22.5487, 21.0354) (-22.5608, 21.0406) (-22.5729, 21.0458) (-22.585, 21.051) (-22.5972, 21.0562) (-22.6094, 21.0614) (-22.6217, 21.0666) (-22.6339, 21.0718) (-22.6462, 21.077) (-22.6586, 21.0822) (-22.671, 21.0873) (-22.6834, 21.0925) (-22.6934, 21.0967) (-22.7009, 21.0998) (-22.7059, 21.1018) (-22.7084, 21.1029) knots 0 0 0 0 0 0 0.00416667 0.00833333 0.0125 0.01666667 0.02083333 0.025 0.02916667 0.03333333 0.0375 0.04166667 0.04583333 0.05 0.05416667 0.05833333 0.0625 0.06666667 0.07083333 0.075 0.07916667 0.08333333 0.0875 0.09166667 0.09583333 0.1 0.10416667 0.10833333 0.1125 0.11666667 0.12083333 0.125 0.12916667 0.13333333 0.1375 0.14166667 0.14583333 0.15 0.15416667 0.15833333 0.1625 0.16666667 0.17083333 0.175 0.17916667 0.18333333 0.1875 0.19166667 0.19583333 0.2 0.20416667 0.20833333 0.2125 0.21666667 0.22083333 0.225 0.22916667 0.23333333 0.2375 0.24166667 0.24583333 0.25 0.25416667 0.25833333 0.2625 0.26666667 0.27083333 0.275 0.27916667 0.28333333 0.2875 0.29166667 0.29583333 0.3 0.30416667 0.30833333 0.3125 0.31666667 0.32083333 0.325 0.32916667 0.33333333 0.3375 0.34166667 0.34583333 0.35 0.35416667 0.35833333 0.3625 0.36666667 0.37083333 0.375 0.37916667 0.38333333 0.3875 0.39166667 0.39583333 0.4 0.40416667 0.40833333 0.4125 0.41666667 0.42083333 0.425 0.42916667 0.43333333 0.4375 0.44166667 0.44583333 0.45 0.45416667 0.45833333 0.4625 0.46666667 0.47083333 0.475 0.47916667 0.48333333 0.4875 0.49166667 0.49583333 0.5 0.50416667 0.50833333 0.5125 0.51666667 0.52083333 0.525 0.52916667 0.53333333 0.5375 0.54166667 0.54583333 0.55 0.55416667 0.55833333 0.5625 0.56666667 0.57083333 0.575 0.57916667 0.58333333 0.5875 0.59166667 0.59583333 0.6 0.60416667 0.60833333 0.6125 0.61666667 0.62083333 0.625 0.62916667 0.63333333 0.6375 0.64166667 0.64583333 0.65 0.65416667 0.65833333 0.6625 0.66666667 0.67083333 0.675 0.67916667 0.68333333 0.6875 0.69166667 0.69583333 0.7 0.70416667 0.70833333 0.7125 0.71666667 0.72083333 0.725 0.72916667 0.73333333 0.7375 0.74166667 0.74583333 0.75 0.75416667 0.75833333 0.7625 0.76666667 0.77083333 0.775 0.77916667 0.78333333 0.7875 0.79166667 0.79583333 0.8 0.80416667 0.80833333 0.8125 0.81666667 0.82083333 0.825 0.82916667 0.83333333 0.8375 0.84166667 0.84583333 0.85 0.85416667 0.85833333 0.8625 0.86666667 0.87083333 0.875 0.87916667 0.88333333 0.8875 0.89166667 0.89583333 0.9 0.90416667 0.90833333 0.9125 0.91666667 0.92083333 0.925 0.92916667 0.93333333 0.9375 0.94166667 0.94583333 0.95 0.95416667 0.95833333 0.9625 0.96666667 0.97083333 0.975 0.97916667 0.98333333 0.9875 0.99166667 0.99583333 1 1 1 1 1 1